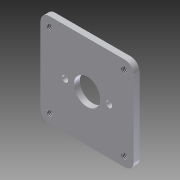
# Autodesk Inventor part: BD gearbox mount top plate
Saved by Autodesk Inventor 2012 (Build 160160000, 160)
## iProperties
Created: 2012-07-04
Part Number: BD gearbox mount top plate
Material: Default
Document SubType Name: Modeling
Designer: Bruce
Density: 1 g/cm^3
Author: Bruce
Autodesk Inventor part; units mm, degrees
ref_plane "YZ Plane" through (0, 0, 0) normal (1, 0, 0) x (0, 1, 0)
ref_plane "XZ Plane" through (0, 0, 0) normal (0, 1, 0) x (-1, 0, 0)
ref_plane "XY Plane" through (0, 0, 0) normal (0, 0, 1) x (1, 0, 0)
sketch "Sketch1" plane through (0, 0, 0) normal (0, 0, 1) x (1, 0, 0)
  line L0 (-13, 12) -> (13, 12)
  line L1 (13, 12) -> (13, -12)
  line L2 (13, -12) -> (-13, -12)
  line L3 (-13, -12) -> (-13, 12)
  line L4 (-13, 3.25) -> (-15, 3.25)
  line L5 (-15, 3.25) -> (-15, -3.25)
  line L6 (-15, -3.25) -> (-13, -3.25)
  line L7 (-13, -3.25) -> (-13, 3.25)
  line L8 (13, 3.25) -> (15, 3.25)
  line L9 (15, 3.25) -> (15, -3.25)
  line L10 (15, -3.25) -> (13, -3.25)
  line L11 (13, -3.25) -> (13, 3.25)
  line L12 (-25.4, 25.4) -> (25.4, 25.4)
  line L13 (25.4, 25.4) -> (25.4, -25.4)
  line L14 (25.4, -25.4) -> (-25.4, -25.4)
  line L15 (-25.4, -25.4) -> (-25.4, 25.4)
  arc A0 (6.3617, 3.25) -> (-6.3617, 3.25) centre (0, 0) ccw
  circle A1 centre (-3, 12) radius 1.5
  line L16 (-13, 8) -> (-9, 12)
  line L17 (9, 12) -> (13, 8)
  line L18 (13, -8) -> (9, -12)
  line L19 (-13, -8) -> (-9, -12)
  line L20 (-14, 3.25) -> (14, 3.25)
  line L21 (-14, -3.25) -> (-6.3617, -3.25)
  arc A2 (6.3617, -3.25) -> (6.3617, 3.25) centre (0, 0) ccw
  arc A3 (-6.3617, 3.25) -> (-6.3617, -3.25) centre (0, 0) ccw
  arc A4 (-6.3617, -3.25) -> (6.3617, -3.25) centre (0, 0) ccw
  line L22 (-6.3617, -3.25) -> (14, -3.25)
  line L23 (-15, 3.25) -> (15, 3.25)
  line L24 (15, 3.25) -> (15, -3.25)
  line L25 (15, -3.25) -> (-15, -3.25)
  line L26 (-15, -3.25) -> (-15, 3.25)
  point P0 (-20.32, 20.32)
  point P1 (20.32, 20.32)
  point P2 (20.32, -20.32)
  point P3 (-20.32, -20.32)
  point P4 (-12, 0)
  point P5 (12, 0)
  dimension "d53" = 3.302
  dimension "d0" = 24
  dimension "d1" = 12
  dimension "d2" = 26
  dimension "d3" = 13
  dimension "d4" = 2
  dimension "d5" = 6.5
  dimension "d6" = 3.25
  dimension "d7" = 2
  dimension "d8" = 14.2875
  dimension "d9" = 50.8
  dimension "d10" = 25.4
  dimension "d11" = 50.8
  dimension "d12" = 25.4
  dimension "d13" = 3
  dimension "d14" = 10
  dimension "d15" = 4
  dimension "d16" = 4
  dimension "d17" = 4
  dimension "d18" = 4
  dimension "d19" = 4
  dimension "d20" = 5.08
  dimension "d21" = 5.08
  dimension "d22" = 5.08
  dimension "d23" = 5.08
  dimension "d34" = 40.64
  dimension "d35" = 40.64
  dimension "d61" = 12
  dimension "d62" = 12
  constraints: 54 end point, 14 point on line, 12 parallel, 9 perpendicular, 8 point on circle, 6 horizontal alignment, 5 centre point, 5 horizontal, 4 midpoint, 2 vertical alignment, 1 coincident, 1 collinear
  measures "d0" distance between parallel lines of L2 L0
  measures "d1" distance from line of L0 point (0, 0)
  measures "d2" distance of L1.end L2.end
  measures "d3" distance from line of L1 point (0, 0)
  measures "d4" distance between parallel lines of L3 L5
  measures "d5" distance of L4.end L5.end
  measures "d6" distance from line of L4 point (0, 0)
  measures "d7" distance between parallel lines of L11 L9
  measures "d8" diameter of A0
  measures "d9" distance of L12.end L13.end
  measures "d10" distance from line of L12 point (0, 0)
  measures "d11" distance of L13.end L14.end
  measures "d12" distance from line of L13 point (0, 0)
  measures "d13" diameter of A1
  measures "d14" distance from line of A1.centre L3
  measures "d15" distance of L0.start L16.end
  measures "d16" distance of L16.start L0.start
  measures "d17" distance from line of L17.start L1
  measures "d18" distance of L2.end L19.start
  measures "d19" distance of L1.end L18.start
  measures "d20" distance from line of point (-20.32, 20.32) L12
  measures "d21" distance from line of L15 point (-20.32, 20.32)
  measures "d22" distance from line of L14 point (-20.32, -20.32)
  measures "d23" distance from line of point (20.32, 20.32) L13
  measures "d34" distance of point (20.32, 20.32) point (-20.32, 20.32)
  measures "d35" distance of point (-20.32, 20.32) point (-20.32, -20.32)
  measures "d61" distance of point (-12, 0) point (0, 0)
  measures "d62" distance of point (12, 0) A0.centre
extrude "Extrusion1" add sketch "Sketch1" against normal blind 3.175 contours L0 L16 L3 | L0 A1 L17 L1 L20 A0 L3 L16 | A1 L0 | L0 A1 | L20 A3 L21 L3 | L3 L6 L5 L4 | L21 A4 L22 L1 L18 L2 L19 L3 | A0 L20 | L20 A2 L22 A3 | L0 L1 L17 | L19 L2 L3 | L22 A4 | L20 L1 L22 A2 | L8 L9 L10 L1 | L18 L1 L2 | L12 L13 L14 L15
fillet "Fillet2" radius 4.7625 4 edges at (25.4, 25.4, -1.5875) (25.4, -25.4, -1.5875) (-25.4, 25.4, -1.5875) (-25.4, -25.4, -1.5875)
hole "Hole2" at (-20.32, 20.32, 0) at (20.32, 20.32, 0) at (20.32, -20.32, 0) at (-20.32, -20.32, 0) direction (0, 0, -1) diameter 3.302 end through all thread size "8-32 UNC" class "2B" standard "ANSI Unified Screw Threads"
extrude "Extrusion6" cut sketch "Sketch1" against normal through all contours A0 L20 | L20 A2 L22 A3 | L22 A4
hole "Hole3" at (-12, 0, 0) at (12, 0, 0) direction (0, 0, -1) diameter 3.3274 end through all
equation "\"d1\" = 0.5 * d0"
equation "\"d3\" = 0.5 * d2"
equation "\"d6\" = 0.5 * d5"
equation "\"d7\" = d4"
equation "\"d10\" = 0.5 * d9"
equation "\"d12\" = 0.5 * d11"
equation "\"d16\" = d15"
equation "\"d17\" = d15"
equation "\"d18\" = d15"
equation "\"d19\" = d15"
equation "\"d22\" = d21"
equation "\"d23\" = d21"
equation "\"d62\" = d61"
body "Solid1"
